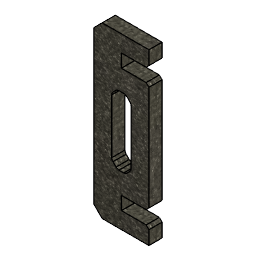
Ensamblaje Blimp CARTON PLUMA (Autodesk Fusion 360 archive; units mm, degrees)
design "SOPORTE INFERIOR"
Autodesk Fusion 360 part; units mm, degrees
(part 1 of 5)
sketch "Boceto1" plane through (0, 0, 0) normal (0, 1, 0) x (1, 0, 0)
  line L0 (3, 0) -> (20, 0)
  line L1 (20, 0) -> (20, -6)
  line L2 (20, -6) -> (10, -6)
  line L3 (10, -6) -> (10, -10.8)
  line L4 (10, -10.8) -> (20, -10.8)
  line L5 (20, -10.8) -> (20, -30.8)
  line L6 (20, -30.8) -> (0, -30.8)
  line L7 (0, -30.8) -> (0, -3)
  line L8 (3, 0) -> (0, -3)
  line L9 (6.5, -30.8) -> (6.5, -20.9213)
  line L10 (9.1213, -18.3) -> (10.8787, -18.3)
  line L11 (13.5, -20.9213) -> (13.5, -30.8)
  line L12 (6.9393, -19.8607) -> (8.0607, -18.7393)
  line L13 (11.9393, -18.7393) -> (13.0607, -19.8607)
  arc A0 (6.9393, -19.8607) -> (6.5, -20.9213) centre (8, -20.9213) ccw
  arc A1 (9.1213, -18.3) -> (8.0607, -18.7393) centre (9.1213, -19.8) ccw
  arc A2 (11.9393, -18.7393) -> (10.8787, -18.3) centre (10.8787, -19.8) ccw
  arc A3 (13.5, -20.9213) -> (13.0607, -19.8607) centre (12, -20.9213) ccw
  line L14 (13.5, -40.6787) -> (13.5, -30.8)
  arc A4 (13.0607, -41.7393) -> (13.5, -40.6787) centre (12, -40.6787) ccw
  line L15 (11.9393, -42.8607) -> (13.0607, -41.7393)
  arc A5 (10.8787, -43.3) -> (11.9393, -42.8607) centre (10.8787, -41.8) ccw
  line L16 (9.1213, -43.3) -> (10.8787, -43.3)
  arc A6 (8.0607, -42.8607) -> (9.1213, -43.3) centre (9.1213, -41.8) ccw
  line L17 (6.9393, -41.7393) -> (8.0607, -42.8607)
  arc A7 (6.5, -40.6787) -> (6.9393, -41.7393) centre (8, -40.6787) ccw
  line L18 (6.5, -30.8) -> (6.5, -40.6787)
  line L19 (20, -50.8) -> (20, -30.8)
  line L20 (0, -30.8) -> (0, -58.6)
  line L21 (10, -50.8) -> (20, -50.8)
  line L22 (20, -55.6) -> (10, -55.6)
  line L23 (10, -55.6) -> (10, -50.8)
  line L24 (20, -61.6) -> (20, -55.6)
  line L25 (3, -61.6) -> (20, -61.6)
  line L26 (3, -61.6) -> (0, -58.6)
  point P0 (6.5, -18.3)
  point P1 (13.5, -18.3)
  point P2 (6.5, -20.3)
  point P3 (8.5, -18.3)
  point P4 (11.5, -18.3)
  point P5 (13.5, -20.3)
  dimension "d1" = 4.8
  dimension "d2" = 40
  dimension "d3" = 6
  dimension "d4" = 20
  dimension "d5" = 10
  dimension "d6" = 3
  dimension "d7" = 3
  dimension "d8" = 7
  dimension "d10" = 7.5
  dimension "d11" = 6.5
  dimension "d12" = 2
  dimension "d13" = 2
  dimension "d14" = 2
  dimension "d15" = 2
  dimension "d16" = 1.5
  constraint horizontal L0
  constraint perpendicular L0 L1
  constraint perpendicular L1 L2
  constraint perpendicular L2 L3
  constraint perpendicular L1 L4
  constraint perpendicular L4 L5
  constraint perpendicular L1 L6
  constraint perpendicular L0 L7
  constraint coincident L1 L4.end
  constraint coincident origin L0
  constraint coincident origin L7
  constraint coincident L6 L9.start
  constraint perpendicular L6 L9
  constraint perpendicular L9 L10
  constraint coincident L6 L11.end
  constraint perpendicular L6 L11
  constraint coincident P0 L9
  constraint coincident P0 L10
  constraint coincident P1 L10
  constraint coincident P1 L11
  constraint coincident P2 L12
  constraint coincident L9 P2
  constraint tangent L12 A0
  constraint tangent L9 A0
  constraint coincident P3 L12
  constraint coincident L10 P3
  constraint tangent L12 A1
  constraint tangent L10 A1
  constraint equal A0 A1
  constraint coincident P4 L13
  constraint coincident L10 P4
  constraint tangent L13 A2
  constraint tangent L10 A2
  constraint equal A0 A2
  constraint coincident P5 L13
  constraint coincident L11 P5
  constraint tangent L13 A3
  constraint tangent L11 A3
  constraint equal A0 A3
  constraint symmetric L0.end L6 L24.start
  constraint symmetric L1.end L6 L22.start
  constraint symmetric L2.end L6 L22.end
  constraint symmetric L3.end L6 L21.start
  constraint symmetric L4.end L6 L19.start
  constraint symmetric L5.end L6 L19.end
  constraint symmetric L7.start L6 L20.start
  constraint symmetric L6 L0.start L25.start
  constraint symmetric L6 L7.end L20.end
  constraint symmetric L6 L9.start L18.start
  constraint symmetric L6 L11.end L14.end
  constraint symmetric L6 L12.start L17.start
  constraint symmetric L6 L9.end A7.start
  constraint symmetric L6 A0 A7
  constraint symmetric L6 L12.end A6.start
  constraint symmetric L6 L10.start L16.start
  constraint symmetric L6 A1 A6
  constraint symmetric L6 L13.start L15.start
  constraint symmetric L6 L10.end A5.start
  constraint symmetric L6 A2 A5
  constraint symmetric L6 L13.end A4.start
  constraint symmetric L6 L11.start L14.start
  constraint symmetric L6 A3 A4
  measures "d1" distance of L2.end L3.end
  measures "d3" distance of L0 L2
  measures "d4" distance of origin L0.end
  measures "d5" distance of L3 L7
  measures "d6" distance of origin L0.start
  measures "d7" distance of origin L7.end
  measures "d8" distance of P0 P1
  measures "d10" distance of L4 L10
  measures "d11" distance of L7 L9
  measures "d12" distance of P0 P2
  measures "d13" distance of P0 P3
  measures "d14" distance of P1 P4
  measures "d15" distance of P1 P5
  measures "d16" radius of A0
extrude "Extruir1" add sketch "Boceto1" along normal blind 4.8 contours L0 L1 L2 L3 L4 L5 L6 L7 L8 L9 L10 L11 L12 L13 A0 A1 A2 A3 | L6 L14 A4 L15 A5 L16 A6 L17 A7 L18 L19 L20 L21 L22 L23 L24 L25 L26
sketch "Boceto2" plane through (0, 0, 0) normal (0, -1, 0) x (1, 0, 0)
  arc A0 (6.5, 20.9213) -> (6.9393, 19.8607) centre (8, 20.9213) ccw
  line L0 (6.5, 20.9213) -> (6.5, 40.6787)
  arc A1 (6.9393, 41.7393) -> (6.5, 40.6787) centre (8, 40.6787) ccw
  line L1 (6.9393, 41.7393) -> (8.0607, 42.8607)
  arc A2 (9.1213, 43.3) -> (8.0607, 42.8607) centre (9.1213, 41.8) ccw
  line L2 (9.1213, 43.3) -> (10.8787, 43.3)
  arc A3 (11.9393, 42.8607) -> (10.8787, 43.3) centre (10.8787, 41.8) ccw
  line L3 (11.9393, 42.8607) -> (13.0607, 41.7393)
  arc A4 (13.5, 40.6787) -> (13.0607, 41.7393) centre (12, 40.6787) ccw
  line L4 (13.5, 40.6787) -> (13.5, 20.9213)
  arc A5 (13.0607, 19.8607) -> (13.5, 20.9213) centre (12, 20.9213) ccw
  line L5 (13.0607, 19.8607) -> (11.9393, 18.7393)
  arc A6 (10.8787, 18.3) -> (11.9393, 18.7393) centre (10.8787, 19.8) ccw
  line L6 (10.8787, 18.3) -> (9.1213, 18.3)
  arc A7 (8.0607, 18.7393) -> (9.1213, 18.3) centre (9.1213, 19.8) ccw
  line L7 (8.0607, 18.7393) -> (6.9393, 19.8607)
  line L8 (20, 55.6) -> (20, 61.6)
  line L9 (20, 61.6) -> (3, 61.6)
  line L10 (3, 61.6) -> (0, 58.6)
  line L11 (0, 58.6) -> (0, 3)
  line L12 (0, 3) -> (3, 0)
  line L13 (3, 0) -> (20, 0)
  line L14 (20, 0) -> (20, 6)
  line L15 (20, 6) -> (10, 6)
  line L16 (10, 6) -> (10, 10.8)
  line L17 (10, 10.8) -> (20, 10.8)
  line L18 (20, 10.8) -> (20, 50.8)
  line L19 (20, 50.8) -> (10, 50.8)
  line L20 (10, 50.8) -> (10, 55.6)
  line L21 (10, 55.6) -> (20, 55.6)
chamfer "Chaflán1" distance 1 angle 45 4 edges at (20, 2.4, 50.8) (20, 2.4, 55.6) (20, 2.4, 6) (20, 2.4, 10.8)
sketch "Boceto3" plane through (0, 0, 0) normal (0, -1, 0) x (1, 0, 0)
  arc A0 (6.5, 20.9213) -> (6.9393, 19.8607) centre (8, 20.9213) ccw
  line L0 (6.5, 20.9213) -> (6.5, 40.6787)
  arc A1 (6.9393, 41.7393) -> (6.5, 40.6787) centre (8, 40.6787) ccw
  line L1 (6.9393, 41.7393) -> (8.0607, 42.8607)
  arc A2 (9.1213, 43.3) -> (8.0607, 42.8607) centre (9.1213, 41.8) ccw
  line L2 (9.1213, 43.3) -> (10.8787, 43.3)
  arc A3 (11.9393, 42.8607) -> (10.8787, 43.3) centre (10.8787, 41.8) ccw
  line L3 (11.9393, 42.8607) -> (13.0607, 41.7393)
  arc A4 (13.5, 40.6787) -> (13.0607, 41.7393) centre (12, 40.6787) ccw
  line L4 (13.5, 40.6787) -> (13.5, 20.9213)
  arc A5 (13.0607, 19.8607) -> (13.5, 20.9213) centre (12, 20.9213) ccw
  line L5 (13.0607, 19.8607) -> (11.9393, 18.7393)
  arc A6 (10.8787, 18.3) -> (11.9393, 18.7393) centre (10.8787, 19.8) ccw
  line L6 (10.8787, 18.3) -> (9.1213, 18.3)
  arc A7 (8.0607, 18.7393) -> (9.1213, 18.3) centre (9.1213, 19.8) ccw
  line L7 (8.0607, 18.7393) -> (6.9393, 19.8607)
  line L8 (19, 10.8) -> (20, 11.8)
  line L9 (20, 11.8) -> (20, 49.8)
  line L10 (20, 49.8) -> (19, 50.8)
  line L11 (19, 50.8) -> (10, 50.8)
  line L12 (10, 50.8) -> (10, 55.6)
  line L13 (10, 55.6) -> (19, 55.6)
  line L14 (19, 55.6) -> (20, 56.6)
  line L15 (20, 56.6) -> (20, 61.6)
  line L16 (20, 61.6) -> (3, 61.6)
  line L17 (3, 61.6) -> (0, 58.6)
  line L18 (0, 58.6) -> (0, 3)
  line L19 (0, 3) -> (3, 0)
  line L20 (3, 0) -> (20, 0)
  line L21 (20, 0) -> (20, 5)
  line L22 (20, 5) -> (19, 6)
  line L23 (19, 6) -> (10, 6)
  line L24 (10, 6) -> (10, 10.8)
  line L25 (10, 10.8) -> (19, 10.8)
equation "d7 = d6"
equation "d13 = d12"
equation "d15 = d14"

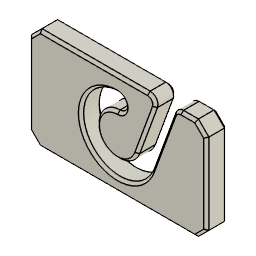
design "SOPORTE PEGADO"
Autodesk Fusion 360 part; units mm, degrees
sketch "Boceto1" plane through (0, 0, 0) normal (0, 1, 0) x (1, 0, 0)
  line L0 (-15, 9.5) -> (15, 9.5)
  line L1 (17, 7.5) -> (17, -8)
  line L2 (-17, -8) -> (-17, 7.5)
  arc A0 (0, -7) -> (0, -4) centre (0, -5.5) ccw
  line L3 (0, -1.75) -> (0, -22.5)
  line L4 (3.7588, 1.3681) -> (7.1637, -7.987)
  line L5 (6.5778, 2.3941) -> (10.7297, -9.013)
  arc A1 (6.5778, 2.3941) -> (0, -7) centre (0, 0) ccw
  arc A2 (3.7588, 1.3681) -> (0, -4) centre (0, 0) ccw
  line L6 (15, -10) -> (12.1393, -10)
  line L7 (5.7542, -10) -> (-15, -10)
  line L8 (-17, -8) -> (-15, -10)
  line L9 (-15, 9.5) -> (-17, 7.5)
  line L10 (15, 9.5) -> (17, 7.5)
  line L11 (17, -8) -> (15, -10)
  arc A3 (5.7542, -10) -> (7.1637, -7.987) centre (5.7542, -8.5) ccw
  arc A4 (10.7297, -9.013) -> (12.1393, -10) centre (12.1393, -8.5) ccw
  point P0 (-17, 9.5)
  point P1 (17, 9.5)
  point P2 (17, -10)
  point P3 (-17, -10)
  dimension "d1" = 8
  dimension "d2" = 14
  dimension "d4" = 10
  dimension "d5" = 9.5
  dimension "d7" = 1.5
  dimension "d8" = 20
  dimension "d9" = 34
  dimension "d10" = 17
  dimension "d11" = 2
  dimension "d12" = 2
  dimension "d13" = 2
  dimension "d14" = 2
  dimension "d15" = 2
  dimension "d16" = 2
  dimension "d17" = 2
  dimension "d18" = 2
  dimension "d19" = 1.5
  constraint coincident A1.centre A2.centre
  constraint concentric A1 A2
  constraint horizontal L0
  constraint vertical L1
  constraint horizontal L6
  constraint vertical L2
  constraint coincident A0.start L3
  constraint coincident A0.end L3
  constraint tangent L4 A2
  constraint parallel L4 L5
  constraint tangent L5 A1
  constraint collinear L6 L7
  constraint coincident P3 L2
  constraint coincident P3 L7
  constraint coincident P0 L0
  constraint coincident P0 L2
  constraint coincident P1 L0
  constraint coincident P1 L1
  constraint coincident P2 L1
  constraint coincident P2 L6
  constraint tangent L4 A3
  constraint tangent L7 A3
  constraint tangent L5 A4
  constraint tangent L6 A4
  constraint equal A3 A4
  measures "d1" diameter of A2
  measures "d2" diameter of A1
  measures "d4" distance of A1.centre L7
  measures "d5" distance of A1.centre L0
  measures "d7" radius of A0
  measures "d8" angle of L3 L4
  measures "d9" distance of L1 L2
  measures "d10" distance of A1.centre L2
  measures "d11" distance of P3 L2.start
  measures "d12" distance of P3 L7.end
  measures "d13" distance of P0 L0.start
  measures "d14" distance of P0 L2.end
  measures "d15" distance of P1 L0.end
  measures "d16" distance of P1 L1.start
  measures "d17" distance of P2 L1.end
  measures "d18" distance of P2 L6.start
  measures "d19" radius of A3
extrude "Extruir1" add sketch "Boceto1" along normal blind 4 contours L0 L1 L2 L3 L5 A1 L6 L7 L8 L9 L10 L11 A4 | A0 L3 L4 A2 L7 A3
chamfer "Chaflán1" distance 0.5 angle 45 2 faces at (13.5259, 0, -0.6314) (13.5259, 4, -0.6314)
equation "d10 = d9 / 2"
equation "d12 = d11"
equation "d14 = d13"
equation "d16 = d15"
equation "d18 = d17"

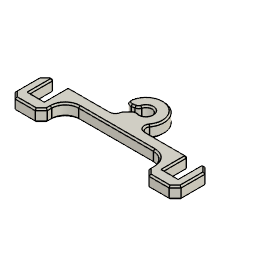
design "SOPORTE IMPRESO GLOBO"
Autodesk Fusion 360 part; units mm, degrees
sketch "Boceto1" plane through (0, 0, 0) normal (0, 0, 1) x (1, 0, 0)
  circle A0 centre (0, 0) radius 2
  circle A1 centre (0, 0) radius 6
  line L0 (-20, -6) -> (-20, -14)
  line L1 (-20, -14) -> (-24.75, -14)
  line L2 (-24.75, -14) -> (-24.75, -6)
  line L3 (-24.75, -6) -> (-27.75, -6)
  line L4 (-27.75, -6) -> (-27.75, -18)
  line L5 (-27.75, -18) -> (-17, -18)
  line L6 (0, -18) -> (0, -6)
  line L7 (-17, -6) -> (-17, -10)
  line L8 (-20, -6) -> (-17, -6)
  line L9 (-4.2426, -4.2426) -> (-4.2426, -6)
  line L10 (-5.9088, -1.0419) -> (-1.9696, -0.3473)
  line L11 (-4.2426, -4.2426) -> (-1.4142, -1.4142)
  line L12 (-24.75, -14) -> (-24.75, 6) construction
  line L13 (0, 6) -> (-24.75, 6) construction
  line L14 (-17, -6) -> (-4.2426, -6)
  line L15 (-17, -10) -> (0, -10)
  line L16 (-17, -10) -> (-17, -18)
  line L17 (24.75, -14) -> (24.75, -6)
  line L18 (24.75, -6) -> (27.75, -6)
  line L19 (27.75, -6) -> (27.75, -18)
  line L20 (27.75, -18) -> (17, -18)
  line L21 (20, -14) -> (24.75, -14)
  line L22 (20, -6) -> (20, -14)
  line L23 (20, -6) -> (17, -6)
  line L24 (17, -6) -> (4.2426, -6)
  line L25 (17, -10) -> (0, -10)
  line L26 (17, -10) -> (17, -18)
  line L27 (4.2426, -4.2426) -> (4.2426, -6)
  dimension "d1" = 4
  dimension "d2" = 4
  dimension "d3" = 4.75
  dimension "d4" = 3
  dimension "d5" = 4
  dimension "d6" = 8
  dimension "d7" = 45
  dimension "d8" = 35
  dimension "d9" = 20
  dimension "d11" = 3
  dimension "d12" = 4
  dimension "d22" = 40
  constraint coincident A0.centre A1.centre
  constraint perpendicular L0 L1
  constraint perpendicular L1 L2
  constraint perpendicular L2 L3
  constraint perpendicular L3 L4
  constraint perpendicular L2 L5
  constraint coincident A1 L6.end
  constraint perpendicular L5 L6
  constraint coincident A0.centre L6
  constraint perpendicular L7 L8
  constraint coincident L2.end L8
  constraint horizontal L8
  constraint horizontal L5
  constraint coincident A1 L9.start
  constraint perpendicular L8 L9
  constraint coincident A1 L10.start
  constraint coincident A0 L10.end
  constraint coincident A0.centre L10
  constraint coincident A0 L11.end
  constraint coincident A0.centre L11
  constraint coincident A1 L13.start
  constraint perpendicular L12 L13
  constraint tangent A1 L13
  constraint coincident L12.end L13.end
  constraint coincident L1 L2.start
  constraint vertical L12
  constraint coincident L1.end L2.start
  constraint perpendicular L9 L14
  constraint perpendicular L9 L15
  constraint perpendicular L5 L16
  constraint coincident L6 L15.end
  constraint symmetric L0.start L6 L22.start
  constraint symmetric L0.end L6 L21.start
  constraint symmetric L1.end L6 L17.start
  constraint symmetric L2.end L6 L17.end
  constraint symmetric L3.end L6 L18.end
  constraint symmetric L4.end L6 L19.end
  constraint symmetric L6 L7.start L23.end
  constraint symmetric L6 L9.start L27.start
  constraint symmetric L6 L9.end L24.end
  constraint symmetric L6 L7.end L25.start
  constraint symmetric L6 L15.end L25.end
  constraint symmetric L6 L5.end L20.end
  measures "d1" diameter of A0
  measures "d2" distance of A0
  measures "d3" distance of L0.end L1.end
  measures "d4" distance of L2.end L3.end
  measures "d5" distance of L1 L5
  measures "d6" distance of L1.end L2.end
  measures "d7" angle of L6 L11
  measures "d8" angle of L10 L11
  measures "d9" distance of L1.end L12.end
  measures "d11" distance of L0.start L7.start
  measures "d12" distance of L14 L15
extrude "Extruir1" add sketch "Boceto1" along normal blind 4 contours A0 A1 L10 L11 | A1 L6 L7 L9 L14 L15 | A1 L6 L17 L18 L19 L20 L21 L22 L23 L24 L25 L26 L27 | L0 L1 L2 L3 L4 L5 L7 L8 L16 picked at (-4.6252, -0.5238)
fillet "Empalme1" radius 4.5 2 edges at (-17, -10, 2) (17, -10, 2)
fillet "Empalme2" radius 1.5 7 edges at (-1.4142, -1.4142, 2) (-1.9696, -0.3473, 2) (-5.9088, -1.0419, 2) (-4.2426, -4.2426, 2) (-4.2426, -6, 2) (4.2426, -6, 2) (4.2426, -4.2426, 2)
chamfer "Chaflán1" distance 0.5 angle 45 4 edges at (-20, -6, 2) (-24.75, -6, 2) (20, -6, 2) (24.75, -6, 2)
chamfer "Chaflán2" distance 2 angle 45 6 edges at (27.75, -6, 2) (27.75, -18, 2) (17, -18, 2) (-17, -18, 2) (-27.75, -18, 2) (-27.75, -6, 2)
chamfer "Chaflán3" distance 0.5 angle 45 2 faces at (-12.5735, -7.3333, 4) (-12.5735, -7.3333, 0)
equation "d11 = d4"

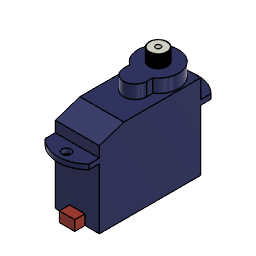
design "MINI SERVO"
Autodesk Fusion 360 part; units mm, degrees
sketch "Boceto1" plane through (0, 0, 0) normal (0, 0, 1) x (1, 0, 0)
  line L0 (0, 0) -> (8.6, 0)
  line L1 (8.6, 0) -> (8.6, 19.8)
  line L2 (8.6, 19.8) -> (0, 19.8)
  line L3 (0, 19.8) -> (0, 0)
  dimension "d1" = 8.6
  dimension "d2" = 19.8
  constraint horizontal L0
  constraint vertical L1
  constraint horizontal L2
  constraint vertical L3
  constraint coincident L0.start L3.end
  measures "d1" distance of L0.start L0.end
  measures "d2" distance of L0.start L2.end
extrude "Extruir1" add sketch "Boceto1" along normal blind 11.85 makes body 1
sketch "Boceto2" plane through (0, 0, 0) normal (0, -1, 0) x (1, 0, 0)
  line L0 (0, 0) -> (8.6, 0)
  line L1 (8.6, 0) -> (8.6, 11.85)
  line L2 (8.6, 11.85) -> (0, 11.85)
  line L3 (0, 11.85) -> (0, 0)
  line L4 (2.8, 0) -> (5.8, 0)
  line L5 (5.8, 0) -> (5.8, 2)
  line L6 (5.8, 2) -> (2.8, 2)
  line L7 (2.8, 2) -> (2.8, 0)
  dimension "d5" = 3
  dimension "d6" = 2
  dimension "d7" = 2.8
  dimension "d8" = 8.6
  constraint horizontal L4
  constraint vertical L5
  constraint horizontal L6
  constraint vertical L7
  constraint coincident L0 L4.start
  measures "d5" distance of L4.start L4.end
  measures "d6" distance of L4.start L6.end
  measures "d7" distance of L0.start L4.start
  measures "d8" distance of L1.end L2.end
extrude "Extruir2" add sketch "Boceto2" along normal blind 2 separate body contours L0 L4 L5 L6 L7 makes body 2
sketch "Boceto3" plane through (0, 0, 11.85) normal (0, 0, 1) x (-1, 0, 0)
  line L0 (0, -19.8) -> (0, 0)
  line L1 (0, 0) -> (-8.6, 0)
  line L2 (-8.6, 0) -> (-8.6, -19.8)
  line L3 (-8.6, -19.8) -> (0, -19.8)
  line L4 (0, -23.6) -> (-8.6, -23.6)
  line L5 (-8.6, -23.6) -> (-8.6, 3.8)
  line L6 (-8.6, 3.8) -> (0, 3.8)
  line L7 (0, 3.8) -> (0, -23.6)
  circle A0 centre (-4.3, -21.9) radius 0.875
  line L8 (-8.6, -9.9) -> (0, -9.9)
  line L9 (-4.3, -19.8) -> (-4.3, -23.6) construction
  arc A1 (-4.3, -23.6) -> (0, -21.8) centre (-4.3, -17.5639) ccw
  arc A2 (-8.6, -21.8) -> (-4.3, -23.6) centre (-4.3, -17.5639) ccw
  arc A3 (0, 2) -> (-4.3, 3.8) centre (-4.3, -2.2361) ccw
  arc A4 (-4.3, 3.8) -> (-8.6, 2) centre (-4.3, -2.2361) ccw
  circle A5 centre (-4.3, 2.1) radius 0.875
  dimension "d11" = 27.4
  dimension "d12" = 3.8
  dimension "d13" = 1.75
  dimension "d14" = 2.1
  dimension "d15" = 2
  constraint horizontal L4
  constraint vertical L5
  constraint horizontal L6
  constraint vertical L7
  constraint midpoint L5 L8.start
  constraint midpoint L7 L8.end
  constraint coincident L0.start L7
  constraint coincident L2.end L5
  constraint midpoint L3 L9.start
  constraint midpoint L4 L9.end
  constraint coincident A0.centre L9
  constraint tangent L4 A1
  constraint coincident L7 A1.end
  constraint symmetric A1.start L9 A2.end
  constraint symmetric L9 A1.end A2.start
  constraint symmetric L9 A1 A2
  constraint symmetric A0 L8 A5
  constraint symmetric L8 L9.end A3.end
  constraint symmetric L8 A1.end A3.start
  constraint symmetric L8 A1 A3
  constraint symmetric L8 A2.start A4.end
  constraint symmetric L8 A2 A4
  measures "d11" distance of L4.end L5.end
  measures "d12" distance of L3 L4
  measures "d13" diameter of A0
  measures "d14" distance of L3 A0.centre
  measures "d15" distance of L0.start A1.end
extrude "Extruir3" add sketch "Boceto3" along normal blind 0.95 contours L0 L2 L3 L5 L7 L8 | L3 L5 L7 A1 A2 | L0 L1 L2 L5 L7 L8 | L1 L5 L7 A3 A4 bodies 1
sketch "Boceto4" plane through (0, 0, 12.8) normal (0, 0, 1) x (-1, 0, 0)
  circle A0 centre (-4.3, 2.1) radius 0.875
  circle A1 centre (-4.3, -21.9) radius 0.875
  arc A2 (0, 2) -> (-8.6, 2) centre (-4.3, -2.2361) ccw
  line L0 (-8.6, 2) -> (-8.6, -21.8)
  arc A3 (-8.6, -21.8) -> (0, -21.8) centre (-4.3, -17.5639) ccw
  line L1 (0, -21.8) -> (0, 2)
  line L2 (0, 0) -> (-8.6, 0)
  line L3 (-8.6, 0) -> (-8.6, -19.8)
  line L4 (-8.6, -19.8) -> (0, -19.8)
  line L5 (0, -19.8) -> (0, 0)
  dimension "d18" = 19.8
  constraint horizontal L2
  constraint vertical L3
  constraint horizontal L4
  constraint vertical L5
  constraint coincident L0 L3.end
  constraint coincident L2.start L5.end
  measures "d18" distance of L2.end L3.end
extrude "Extruir4" add sketch "Boceto4" along normal blind 3.7 contours L0 L1 L2 L3 L4 L5 bodies 1
sketch "Boceto5" plane through (0, 0, 16.5) normal (0, 0, 1) x (-1, 0, 0)
  line L0 (0, -19.8) -> (0, 0)
  line L1 (0, 0) -> (-8.6, 0)
  line L2 (-8.6, 0) -> (-8.6, -19.8)
  line L3 (-8.6, -19.8) -> (0, -19.8)
  circle A0 centre (-4.3, -15.8) radius 4
  line L4 (-4.3, -19.8) -> (-4.3, 0)
  line L5 (-2.05, -11.3) -> (-2.05, -12.4928)
  line L6 (-6.55, -11.3) -> (-6.55, -12.4928)
  arc A1 (-2.05, -11.3) -> (-6.55, -11.3) centre (-4.3, -11.3) ccw
  dimension "d21" = 8
  dimension "d22" = 4.5
  dimension "d23" = 4.5
  constraint tangent L3 A0
  constraint midpoint L3 L4.start
  constraint midpoint L1 L4.end
  constraint coincident A0.centre L4
  constraint coincident A0 L5.end
  constraint tangent L5 A1
  constraint parallel L4 L5
  constraint coincident A0 L6.end
  constraint tangent L6 A1
  constraint parallel L4 L6
  constraint coincident L4 A1.centre
  measures "d21" diameter of A0
  measures "d22" diameter of A1
  measures "d23" distance of A0.centre A1.centre
extrude "Extruir5" add sketch "Boceto5" along normal blind 2.6 contours A0 L4 | A0 L4 | A0 L4 L6 A1 | A0 L4 L5 A1 bodies 1
chamfer "Chaflán1" distance 4.8 distance2 1.6 1 edges at (4.3, 0, 16.5) measured on face at (4.356, 3.0188, 16.5) on bodies 1
sketch "Boceto6" plane through (0, 0, 19.1) normal (0, 0, 1) x (-1, 0, 0)
  arc A0 (-2.05, -11.3) -> (-6.55, -11.3) centre (-4.3, -11.3) ccw
  line L0 (-6.55, -11.3) -> (-6.55, -12.4928)
  arc A1 (-6.55, -12.4928) -> (-2.05, -12.4928) centre (-4.3, -15.8) ccw
  line L1 (-2.05, -12.4928) -> (-2.05, -11.3)
  circle A2 centre (-4.3, -15.8) radius 1.75
  circle A3 centre (-4.3, -15.8) radius 0.5
  line L2 (-4.2713, -17.5498) -> (-4.28, -17.5005)
  line L3 (-4.28, -17.5005) -> (-4.32, -17.5005)
  line L4 (-4.32, -17.5005) -> (-4.3287, -17.5498)
  line L5 (-4.3, -17.5005) -> (-4.3, -15.8) construction
  line L6 (-4.2132, -17.4984) -> (-4.2188, -17.5481)
  line L7 (-4.1733, -17.4959) -> (-4.2132, -17.4984)
  line L8 (-4.1615, -17.5445) -> (-4.1733, -17.4959)
  line L9 (-4.1067, -17.4896) -> (-4.1092, -17.5396)
  line L10 (-4.067, -17.4846) -> (-4.1067, -17.4896)
  line L11 (-4.0522, -17.5324) -> (-4.067, -17.4846)
  line L12 (-4.001, -17.4742) -> (-4.0003, -17.5241)
  line L13 (-3.9617, -17.4667) -> (-4.001, -17.4742)
  line L14 (-3.944, -17.5134) -> (-3.9617, -17.4667)
  line L15 (-3.8965, -17.4521) -> (-3.8926, -17.5019)
  line L16 (-3.8577, -17.4421) -> (-3.8965, -17.4521)
  line L17 (-3.8371, -17.4877) -> (-3.8577, -17.4421)
  line L18 (-3.7935, -17.4235) -> (-3.7866, -17.473)
  line L19 (-3.7555, -17.4111) -> (-3.7935, -17.4235)
  line L20 (-3.732, -17.4553) -> (-3.7555, -17.4111)
  line L21 (-3.6926, -17.3885) -> (-3.6825, -17.4374)
  line L22 (-3.6554, -17.3737) -> (-3.6926, -17.3885)
  line L23 (-3.6292, -17.4163) -> (-3.6554, -17.3737)
  line L24 (-3.594, -17.3472) -> (-3.5809, -17.3954)
  line L25 (-3.5579, -17.3302) -> (-3.594, -17.3472)
  line L26 (-3.529, -17.371) -> (-3.5579, -17.3302)
  line L27 (-3.4983, -17.2998) -> (-3.4822, -17.3471)
  line L28 (-3.4632, -17.2805) -> (-3.4983, -17.2998)
  line L29 (-3.4319, -17.3195) -> (-3.4632, -17.2805)
  line L30 (-3.4057, -17.2465) -> (-3.3866, -17.2927)
  line L31 (-3.3719, -17.2251) -> (-3.4057, -17.2465)
  line L32 (-3.3382, -17.262) -> (-3.3719, -17.2251)
  line L33 (-3.3166, -17.1875) -> (-3.2947, -17.2324)
  line L34 (-3.2843, -17.164) -> (-3.3166, -17.1875)
  line L35 (-3.2483, -17.1987) -> (-3.2843, -17.164)
  line L36 (-3.2315, -17.123) -> (-3.2068, -17.1665)
  line L37 (-3.2006, -17.0975) -> (-3.2315, -17.123)
  line L38 (-3.1626, -17.1299) -> (-3.2006, -17.0975)
  line L39 (-3.1505, -17.0533) -> (-3.1231, -17.0952)
  line L40 (-3.1213, -17.0259) -> (-3.1505, -17.0533)
  line L41 (-3.0813, -17.0559) -> (-3.1213, -17.0259)
  line L42 (-3.0741, -16.9787) -> (-3.0441, -17.0187)
  line L43 (-3.0467, -16.9495) -> (-3.0741, -16.9787)
  line L44 (-3.0048, -16.9769) -> (-3.0467, -16.9495)
  line L45 (-3.0025, -16.8994) -> (-2.9701, -16.9374)
  line L46 (-2.977, -16.8685) -> (-3.0025, -16.8994)
  line L47 (-2.9335, -16.8932) -> (-2.977, -16.8685)
  line L48 (-2.936, -16.8157) -> (-2.9013, -16.8517)
  line L49 (-2.9125, -16.7834) -> (-2.936, -16.8157)
  line L50 (-2.8676, -16.8053) -> (-2.9125, -16.7834)
  line L51 (-2.8749, -16.7281) -> (-2.838, -16.7618)
  line L52 (-2.8535, -16.6943) -> (-2.8749, -16.7281)
  line L53 (-2.8073, -16.7134) -> (-2.8535, -16.6943)
  line L54 (-2.8195, -16.6368) -> (-2.7805, -16.6681)
  line L55 (-2.8002, -16.6017) -> (-2.8195, -16.6368)
  line L56 (-2.7529, -16.6178) -> (-2.8002, -16.6017)
  line L57 (-2.7698, -16.5421) -> (-2.729, -16.571)
  line L58 (-2.7528, -16.506) -> (-2.7698, -16.5421)
  line L59 (-2.7046, -16.5191) -> (-2.7528, -16.506)
  line L60 (-2.7263, -16.4446) -> (-2.6837, -16.4708)
  line L61 (-2.7115, -16.4074) -> (-2.7263, -16.4446)
  line L62 (-2.6626, -16.4175) -> (-2.7115, -16.4074)
  line L63 (-2.6889, -16.3445) -> (-2.6447, -16.368)
  line L64 (-2.6765, -16.3065) -> (-2.6889, -16.3445)
  line L65 (-2.627, -16.3134) -> (-2.6765, -16.3065)
  line L66 (-2.6579, -16.2423) -> (-2.6123, -16.2629)
  line L67 (-2.6479, -16.2035) -> (-2.6579, -16.2423)
  line L68 (-2.5981, -16.2074) -> (-2.6479, -16.2035)
  line L69 (-2.6333, -16.1383) -> (-2.5866, -16.156)
  line L70 (-2.6258, -16.099) -> (-2.6333, -16.1383)
  line L71 (-2.5759, -16.0997) -> (-2.6258, -16.099)
  line L72 (-2.6154, -16.033) -> (-2.5676, -16.0478)
  line L73 (-2.6104, -15.9933) -> (-2.6154, -16.033)
  line L74 (-2.5604, -15.9908) -> (-2.6104, -15.9933)
  line L75 (-2.6041, -15.9267) -> (-2.5555, -15.9385)
  line L76 (-2.6016, -15.8868) -> (-2.6041, -15.9267)
  line L77 (-2.5519, -15.8812) -> (-2.6016, -15.8868)
  line L78 (-2.5995, -15.82) -> (-2.5502, -15.8287)
  line L79 (-2.5995, -15.78) -> (-2.5995, -15.82)
  line L80 (-2.5502, -15.7713) -> (-2.5995, -15.78)
  line L81 (-2.6016, -15.7132) -> (-2.5519, -15.7188)
  line L82 (-2.6041, -15.6733) -> (-2.6016, -15.7132)
  line L83 (-2.5555, -15.6615) -> (-2.6041, -15.6733)
  line L84 (-2.6104, -15.6067) -> (-2.5604, -15.6092)
  line L85 (-2.6154, -15.567) -> (-2.6104, -15.6067)
  line L86 (-2.5676, -15.5522) -> (-2.6154, -15.567)
  line L87 (-2.6258, -15.501) -> (-2.5759, -15.5003)
  line L88 (-2.6333, -15.4617) -> (-2.6258, -15.501)
  line L89 (-2.5866, -15.444) -> (-2.6333, -15.4617)
  line L90 (-2.6479, -15.3965) -> (-2.5981, -15.3926)
  line L91 (-2.6579, -15.3577) -> (-2.6479, -15.3965)
  line L92 (-2.6123, -15.3371) -> (-2.6579, -15.3577)
  line L93 (-2.6765, -15.2935) -> (-2.627, -15.2866)
  line L94 (-2.6889, -15.2555) -> (-2.6765, -15.2935)
  line L95 (-2.6447, -15.232) -> (-2.6889, -15.2555)
  line L96 (-2.7115, -15.1926) -> (-2.6626, -15.1825)
  line L97 (-2.7263, -15.1554) -> (-2.7115, -15.1926)
  line L98 (-2.6837, -15.1292) -> (-2.7263, -15.1554)
  line L99 (-2.7528, -15.094) -> (-2.7046, -15.0809)
  line L100 (-2.7698, -15.0579) -> (-2.7528, -15.094)
  line L101 (-2.729, -15.029) -> (-2.7698, -15.0579)
  line L102 (-2.8002, -14.9983) -> (-2.7529, -14.9822)
  line L103 (-2.8195, -14.9632) -> (-2.8002, -14.9983)
  line L104 (-2.7805, -14.9319) -> (-2.8195, -14.9632)
  line L105 (-2.8535, -14.9057) -> (-2.8073, -14.8866)
  line L106 (-2.8749, -14.8719) -> (-2.8535, -14.9057)
  line L107 (-2.838, -14.8382) -> (-2.8749, -14.8719)
  line L108 (-2.9125, -14.8166) -> (-2.8676, -14.7947)
  line L109 (-2.936, -14.7843) -> (-2.9125, -14.8166)
  line L110 (-2.9013, -14.7483) -> (-2.936, -14.7843)
  line L111 (-2.977, -14.7315) -> (-2.9335, -14.7068)
  line L112 (-3.0025, -14.7006) -> (-2.977, -14.7315)
  line L113 (-2.9701, -14.6626) -> (-3.0025, -14.7006)
  line L114 (-3.0467, -14.6505) -> (-3.0048, -14.6231)
  line L115 (-3.0741, -14.6213) -> (-3.0467, -14.6505)
  line L116 (-3.0441, -14.5813) -> (-3.0741, -14.6213)
  line L117 (-3.1213, -14.5741) -> (-3.0813, -14.5441)
  line L118 (-3.1505, -14.5467) -> (-3.1213, -14.5741)
  line L119 (-3.1231, -14.5048) -> (-3.1505, -14.5467)
  line L120 (-3.2006, -14.5025) -> (-3.1626, -14.4701)
  line L121 (-3.2315, -14.477) -> (-3.2006, -14.5025)
  line L122 (-3.2068, -14.4335) -> (-3.2315, -14.477)
  line L123 (-3.2843, -14.436) -> (-3.2483, -14.4013)
  line L124 (-3.3166, -14.4125) -> (-3.2843, -14.436)
  line L125 (-3.2947, -14.3676) -> (-3.3166, -14.4125)
  line L126 (-3.3719, -14.3749) -> (-3.3382, -14.338)
  line L127 (-3.4057, -14.3535) -> (-3.3719, -14.3749)
  line L128 (-3.3866, -14.3073) -> (-3.4057, -14.3535)
  line L129 (-3.4632, -14.3195) -> (-3.4319, -14.2805)
  line L130 (-3.4983, -14.3002) -> (-3.4632, -14.3195)
  line L131 (-3.4822, -14.2529) -> (-3.4983, -14.3002)
  line L132 (-3.5579, -14.2698) -> (-3.529, -14.229)
  line L133 (-3.594, -14.2528) -> (-3.5579, -14.2698)
  line L134 (-3.5809, -14.2046) -> (-3.594, -14.2528)
  line L135 (-3.6554, -14.2263) -> (-3.6292, -14.1837)
  line L136 (-3.6926, -14.2115) -> (-3.6554, -14.2263)
  line L137 (-3.6825, -14.1626) -> (-3.6926, -14.2115)
  line L138 (-3.7555, -14.1889) -> (-3.732, -14.1447)
  line L139 (-3.7935, -14.1765) -> (-3.7555, -14.1889)
  line L140 (-3.7866, -14.127) -> (-3.7935, -14.1765)
  line L141 (-3.8577, -14.1579) -> (-3.8371, -14.1123)
  line L142 (-3.8965, -14.1479) -> (-3.8577, -14.1579)
  line L143 (-3.8926, -14.0981) -> (-3.8965, -14.1479)
  line L144 (-3.9617, -14.1333) -> (-3.944, -14.0866)
  line L145 (-4.001, -14.1258) -> (-3.9617, -14.1333)
  line L146 (-4.0003, -14.0759) -> (-4.001, -14.1258)
  line L147 (-4.067, -14.1154) -> (-4.0522, -14.0676)
  line L148 (-4.1067, -14.1104) -> (-4.067, -14.1154)
  line L149 (-4.1092, -14.0604) -> (-4.1067, -14.1104)
  line L150 (-4.1733, -14.1041) -> (-4.1615, -14.0555)
  line L151 (-4.2132, -14.1016) -> (-4.1733, -14.1041)
  line L152 (-4.2188, -14.0519) -> (-4.2132, -14.1016)
  line L153 (-4.28, -14.0995) -> (-4.2713, -14.0502)
  line L154 (-4.32, -14.0995) -> (-4.28, -14.0995)
  line L155 (-4.3287, -14.0502) -> (-4.32, -14.0995)
  line L156 (-4.3868, -14.1016) -> (-4.3812, -14.0519)
  line L157 (-4.4267, -14.1041) -> (-4.3868, -14.1016)
  line L158 (-4.4385, -14.0555) -> (-4.4267, -14.1041)
  line L159 (-4.4933, -14.1104) -> (-4.4908, -14.0604)
  line L160 (-4.533, -14.1154) -> (-4.4933, -14.1104)
  line L161 (-4.5478, -14.0676) -> (-4.533, -14.1154)
  line L162 (-4.599, -14.1258) -> (-4.5997, -14.0759)
  line L163 (-4.6383, -14.1333) -> (-4.599, -14.1258)
  line L164 (-4.656, -14.0866) -> (-4.6383, -14.1333)
  line L165 (-4.7035, -14.1479) -> (-4.7074, -14.0981)
  line L166 (-4.7423, -14.1579) -> (-4.7035, -14.1479)
  line L167 (-4.7629, -14.1123) -> (-4.7423, -14.1579)
  line L168 (-4.8065, -14.1765) -> (-4.8134, -14.127)
  line L169 (-4.8445, -14.1889) -> (-4.8065, -14.1765)
  line L170 (-4.868, -14.1447) -> (-4.8445, -14.1889)
  line L171 (-4.9074, -14.2115) -> (-4.9175, -14.1626)
  line L172 (-4.9446, -14.2263) -> (-4.9074, -14.2115)
  line L173 (-4.9708, -14.1837) -> (-4.9446, -14.2263)
  line L174 (-5.006, -14.2528) -> (-5.0191, -14.2046)
  line L175 (-5.0421, -14.2698) -> (-5.006, -14.2528)
  line L176 (-5.071, -14.229) -> (-5.0421, -14.2698)
  line L177 (-5.1017, -14.3002) -> (-5.1178, -14.2529)
  line L178 (-5.1368, -14.3195) -> (-5.1017, -14.3002)
  line L179 (-5.1681, -14.2805) -> (-5.1368, -14.3195)
  line L180 (-5.1943, -14.3535) -> (-5.2134, -14.3073)
  line L181 (-5.2281, -14.3749) -> (-5.1943, -14.3535)
  line L182 (-5.2618, -14.338) -> (-5.2281, -14.3749)
  line L183 (-5.2834, -14.4125) -> (-5.3053, -14.3676)
  line L184 (-5.3157, -14.436) -> (-5.2834, -14.4125)
  line L185 (-5.3517, -14.4013) -> (-5.3157, -14.436)
  line L186 (-5.3685, -14.477) -> (-5.3932, -14.4335)
  line L187 (-5.3994, -14.5025) -> (-5.3685, -14.477)
  line L188 (-5.4374, -14.4701) -> (-5.3994, -14.5025)
  line L189 (-5.4495, -14.5467) -> (-5.4769, -14.5048)
  line L190 (-5.4787, -14.5741) -> (-5.4495, -14.5467)
  line L191 (-5.5187, -14.5441) -> (-5.4787, -14.5741)
  line L192 (-5.5259, -14.6213) -> (-5.5559, -14.5813)
  line L193 (-5.5533, -14.6505) -> (-5.5259, -14.6213)
  line L194 (-5.5952, -14.6231) -> (-5.5533, -14.6505)
  line L195 (-5.5975, -14.7006) -> (-5.6299, -14.6626)
  line L196 (-5.623, -14.7315) -> (-5.5975, -14.7006)
  line L197 (-5.6665, -14.7068) -> (-5.623, -14.7315)
  line L198 (-5.664, -14.7843) -> (-5.6987, -14.7483)
  line L199 (-5.6875, -14.8166) -> (-5.664, -14.7843)
  line L200 (-5.7324, -14.7947) -> (-5.6875, -14.8166)
  line L201 (-5.7251, -14.8719) -> (-5.762, -14.8382)
  line L202 (-5.7465, -14.9057) -> (-5.7251, -14.8719)
  line L203 (-5.7927, -14.8866) -> (-5.7465, -14.9057)
  line L204 (-5.7805, -14.9632) -> (-5.8195, -14.9319)
  line L205 (-5.7998, -14.9983) -> (-5.7805, -14.9632)
  line L206 (-5.8471, -14.9822) -> (-5.7998, -14.9983)
  line L207 (-5.8302, -15.0579) -> (-5.871, -15.029)
  line L208 (-5.8472, -15.094) -> (-5.8302, -15.0579)
  line L209 (-5.8954, -15.0809) -> (-5.8472, -15.094)
  line L210 (-5.8737, -15.1554) -> (-5.9163, -15.1292)
  line L211 (-5.8885, -15.1926) -> (-5.8737, -15.1554)
  line L212 (-5.9374, -15.1825) -> (-5.8885, -15.1926)
  line L213 (-5.9111, -15.2555) -> (-5.9553, -15.232)
  line L214 (-5.9235, -15.2935) -> (-5.9111, -15.2555)
  line L215 (-5.973, -15.2866) -> (-5.9235, -15.2935)
  line L216 (-5.9421, -15.3577) -> (-5.9877, -15.3371)
  line L217 (-5.9521, -15.3965) -> (-5.9421, -15.3577)
  line L218 (-6.0019, -15.3926) -> (-5.9521, -15.3965)
  line L219 (-5.9667, -15.4617) -> (-6.0134, -15.444)
  line L220 (-5.9742, -15.501) -> (-5.9667, -15.4617)
  line L221 (-6.0241, -15.5003) -> (-5.9742, -15.501)
  line L222 (-5.9846, -15.567) -> (-6.0324, -15.5522)
  line L223 (-5.9896, -15.6067) -> (-5.9846, -15.567)
  line L224 (-6.0396, -15.6092) -> (-5.9896, -15.6067)
  line L225 (-5.9959, -15.6733) -> (-6.0445, -15.6615)
  line L226 (-5.9984, -15.7132) -> (-5.9959, -15.6733)
  line L227 (-6.0481, -15.7188) -> (-5.9984, -15.7132)
  line L228 (-6.0005, -15.78) -> (-6.0498, -15.7713)
  line L229 (-6.0005, -15.82) -> (-6.0005, -15.78)
  line L230 (-6.0498, -15.8287) -> (-6.0005, -15.82)
  line L231 (-5.9984, -15.8868) -> (-6.0481, -15.8812)
  line L232 (-5.9959, -15.9267) -> (-5.9984, -15.8868)
  line L233 (-6.0445, -15.9385) -> (-5.9959, -15.9267)
  line L234 (-5.9896, -15.9933) -> (-6.0396, -15.9908)
  line L235 (-5.9846, -16.033) -> (-5.9896, -15.9933)
  line L236 (-6.0324, -16.0478) -> (-5.9846, -16.033)
  line L237 (-5.9742, -16.099) -> (-6.0241, -16.0997)
  line L238 (-5.9667, -16.1383) -> (-5.9742, -16.099)
  line L239 (-6.0134, -16.156) -> (-5.9667, -16.1383)
  line L240 (-5.9521, -16.2035) -> (-6.0019, -16.2074)
  line L241 (-5.9421, -16.2423) -> (-5.9521, -16.2035)
  line L242 (-5.9877, -16.2629) -> (-5.9421, -16.2423)
  line L243 (-5.9235, -16.3065) -> (-5.973, -16.3134)
  line L244 (-5.9111, -16.3445) -> (-5.9235, -16.3065)
  line L245 (-5.9553, -16.368) -> (-5.9111, -16.3445)
  line L246 (-5.8885, -16.4074) -> (-5.9374, -16.4175)
  line L247 (-5.8737, -16.4446) -> (-5.8885, -16.4074)
  line L248 (-5.9163, -16.4708) -> (-5.8737, -16.4446)
  line L249 (-5.8472, -16.506) -> (-5.8954, -16.5191)
  line L250 (-5.8302, -16.5421) -> (-5.8472, -16.506)
  line L251 (-5.871, -16.571) -> (-5.8302, -16.5421)
  line L252 (-5.7998, -16.6017) -> (-5.8471, -16.6178)
  line L253 (-5.7805, -16.6368) -> (-5.7998, -16.6017)
  line L254 (-5.8195, -16.6681) -> (-5.7805, -16.6368)
  line L255 (-5.7465, -16.6943) -> (-5.7927, -16.7134)
  line L256 (-5.7251, -16.7281) -> (-5.7465, -16.6943)
  line L257 (-5.762, -16.7618) -> (-5.7251, -16.7281)
  line L258 (-5.6875, -16.7834) -> (-5.7324, -16.8053)
  line L259 (-5.664, -16.8157) -> (-5.6875, -16.7834)
  line L260 (-5.6987, -16.8517) -> (-5.664, -16.8157)
  line L261 (-5.623, -16.8685) -> (-5.6665, -16.8932)
  line L262 (-5.5975, -16.8994) -> (-5.623, -16.8685)
  line L263 (-5.6299, -16.9374) -> (-5.5975, -16.8994)
  line L264 (-5.5533, -16.9495) -> (-5.5952, -16.9769)
  line L265 (-5.5259, -16.9787) -> (-5.5533, -16.9495)
  line L266 (-5.5559, -17.0187) -> (-5.5259, -16.9787)
  line L267 (-5.4787, -17.0259) -> (-5.5187, -17.0559)
  line L268 (-5.4495, -17.0533) -> (-5.4787, -17.0259)
  line L269 (-5.4769, -17.0952) -> (-5.4495, -17.0533)
  line L270 (-5.3994, -17.0975) -> (-5.4374, -17.1299)
  line L271 (-5.3685, -17.123) -> (-5.3994, -17.0975)
  line L272 (-5.3932, -17.1665) -> (-5.3685, -17.123)
  line L273 (-5.3157, -17.164) -> (-5.3517, -17.1987)
  line L274 (-5.2834, -17.1875) -> (-5.3157, -17.164)
  line L275 (-5.3053, -17.2324) -> (-5.2834, -17.1875)
  line L276 (-5.2281, -17.2251) -> (-5.2618, -17.262)
  line L277 (-5.1943, -17.2465) -> (-5.2281, -17.2251)
  line L278 (-5.2134, -17.2927) -> (-5.1943, -17.2465)
  line L279 (-5.1368, -17.2805) -> (-5.1681, -17.3195)
  line L280 (-5.1017, -17.2998) -> (-5.1368, -17.2805)
  line L281 (-5.1178, -17.3471) -> (-5.1017, -17.2998)
  line L282 (-5.0421, -17.3302) -> (-5.071, -17.371)
  line L283 (-5.006, -17.3472) -> (-5.0421, -17.3302)
  line L284 (-5.0191, -17.3954) -> (-5.006, -17.3472)
  line L285 (-4.9446, -17.3737) -> (-4.9708, -17.4163)
  line L286 (-4.9074, -17.3885) -> (-4.9446, -17.3737)
  line L287 (-4.9175, -17.4374) -> (-4.9074, -17.3885)
  line L288 (-4.8445, -17.4111) -> (-4.868, -17.4553)
  line L289 (-4.8065, -17.4235) -> (-4.8445, -17.4111)
  line L290 (-4.8134, -17.473) -> (-4.8065, -17.4235)
  line L291 (-4.7423, -17.4421) -> (-4.7629, -17.4877)
  line L292 (-4.7035, -17.4521) -> (-4.7423, -17.4421)
  line L293 (-4.7074, -17.5019) -> (-4.7035, -17.4521)
  line L294 (-4.6383, -17.4667) -> (-4.656, -17.5134)
  line L295 (-4.599, -17.4742) -> (-4.6383, -17.4667)
  line L296 (-4.5997, -17.5241) -> (-4.599, -17.4742)
  line L297 (-4.533, -17.4846) -> (-4.5478, -17.5324)
  line L298 (-4.4933, -17.4896) -> (-4.533, -17.4846)
  line L299 (-4.4908, -17.5396) -> (-4.4933, -17.4896)
  line L300 (-4.4267, -17.4959) -> (-4.4385, -17.5445)
  line L301 (-4.3868, -17.4984) -> (-4.4267, -17.4959)
  line L302 (-4.3812, -17.5481) -> (-4.3868, -17.4984)
  dimension "d28" = 3.5
  dimension "d29" = 1
  dimension "d30" = 100
  dimension "d31" = 100
  dimension "d33" = 0.04
  dimension "d34" = 0.05
  dimension "d36" = 360
  constraint concentric A1 A2
  constraint concentric A2 A3
  constraint coincident A2 L2.start
  constraint coincident A2 L4.end
  constraint horizontal L3
  constraint midpoint L3 L5.start
  constraint vertical L5
  constraint coincident A1.centre A2.centre
  measures "d28" diameter of A2
  measures "d29" diameter of A3
  measures "d30" angle of L2 L3
  measures "d31" angle of L3 L4
  measures "d33" distance of L2.end L3.end
  measures "d34" distance of L3.end L4.end
extrude "Extruir6" add sketch "Boceto6" along normal blind 2.5 separate body contours A2 L2 L3 L4 L6 L7 L8 L9 L10 L11 L12 L13 L14 L15 L16 L17 L18 L19 L20 L21 L22 L23 L24 L25 L26 L27 L28 L29 L30 L31 L32 L33 L34 L35 L36 L37 L38 L39 L40 L41 L42 L43 L44 L45 L46 L47 L48 L49 L50 L51 L52 L53 L54 L55 L56 L57 L58 L59 L60 L61 L62 L63 L64 L65 L66 L67 L68 L69 L70 L71 L72 L73 L74 L75 L76 L77 L78 L79 L80 L81 L82 L83 L84 L85 L86 L87 L88 L89 L90 L91 L92 L93 L94 L95 L96 L97 L98 L99 L100 L101 L102 L103 L104 L105 L106 L107 L108 L109 L110 L111 L112 L113 L114 L115 L116 L117 L118 L119 L120 L121 L122 L123 L124 L125 L126 L127 L128 L129 L130 L131 L132 L133 L134 L135 L136 L137 L138 L139 L140 L141 L142 L143 L144 L145 L146 L147 L148 L149 L150 L151 L152 L153 L154 L155 L156 L157 L158 L159 L160 L161 L162 L163 L164 L165 L166 L167 L168 L169 L170 L171 L172 L173 L174 L175 L176 L177 L178 L179 L180 L181 L182 L183 L184 L185 L186 L187 L188 L189 L190 L191 L192 L193 L194 L195 L196 L197 L198 L199 L200 L201 L202 L203 L204 L205 L206 L207 L208 L209 L210 L211 L212 L213 L214 L215 L216 L217 L218 L219 L220 L221 L222 L223 L224 L225 L226 L227 L228 L229 L230 L231 L232 L233 L234 L235 L236 L237 L238 L239 L240 L241 L242 L243 L244 L245 L246 L247 L248 L249 L250 L251 L252 L253 L254 L255 L256 L257 L258 L259 L260 L261 L262 L263 L264 L265 L266 L267 L268 L269 L270 L271 L272 L273 L274 L275 L276 L277 L278 L279 L280 L281 L282 L283 L284 L285 L286 L287 L288 L289 L290 L291 L292 L293 L294 L295 L296 L297 L298 L299 L300 L301 L302 makes body 3
equation "d7 = ( d8 - d5 ) / 2"
equation "d12 = ( d11 - 19.8 mm ) / 2"
equation "d24 = 19.1 mm - 16.5 mm"
equation "d30 = d31"

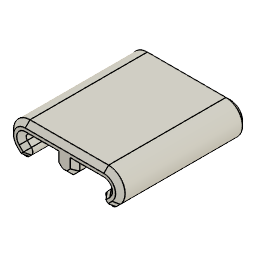
design "SEGUROS MOTORES 2"
Autodesk Fusion 360 part; units mm, degrees
sketch "Boceto1" plane through (0, 0, 0) normal (0, 1, 0) x (1, 0, 0)
  line L0 (-5.4, 0) -> (-6.5464, -1.1464)
  line L1 (-5.4, 0) -> (-3.3228, 0) construction
  line L2 (-6.1929, -2) -> (-1.75, -2)
  line L3 (-1.75, -2) -> (-1.75, 0)
  line L4 (0, -0.3508) -> (0, 0)
  line L5 (-5.4, 0) -> (0, 0)
  arc A0 (-6.5464, -1.1464) -> (-6.1929, -2) centre (-6.1929, -1.5) ccw
  line L6 (0.1, -0.3508) -> (0.1, 0.1)
  line L7 (-5.4414, 0.1) -> (0.1, 0.1)
  line L8 (-5.4414, 0.1) -> (-6.6172, -1.0757)
  arc A1 (-6.6172, -1.0757) -> (-6.1929, -2.1) centre (-6.1929, -1.5) ccw
  line L9 (-6.1929, -2.1) -> (-1.65, -2.1)
  line L10 (-1.65, -2.1) -> (-1.65, 0)
  line L11 (-5.4414, 0.1) -> (-6.8556, 1.5142)
  line L12 (-6.8556, 1.5142) -> (-8.0314, 0.3385)
  line L13 (-6.1929, -4.1) -> (0, -4.1)
  arc A2 (-8.0314, 0.3385) -> (-6.1929, -4.1) centre (-6.1929, -1.5) ccw
  line L14 (5.4414, 0.1) -> (6.8556, 1.5142)
  line L15 (5.4414, 0.1) -> (6.6172, -1.0757)
  arc A3 (6.1929, -2.1) -> (6.6172, -1.0757) centre (6.1929, -1.5) ccw
  line L16 (6.8556, 1.5142) -> (8.0314, 0.3385)
  arc A4 (6.1929, -4.1) -> (8.0314, 0.3385) centre (6.1929, -1.5) ccw
  line L17 (6.1929, -4.1) -> (0, -4.1)
  line L18 (6.1929, -2.1) -> (1.65, -2.1)
  line L19 (1.65, -2.1) -> (1.65, 0)
  line L20 (5.4, 0) -> (0, 0)
  point P0 (-7.4, -2)
  dimension "d1" = 135
  dimension "d2" = 3.5
  dimension "d3" = 2
  dimension "d5" = 10.8
  dimension "d6" = 0.5
  dimension "d7" = 0.1
  dimension "d8" = 2
  dimension "d9" = 2
  constraint horizontal L1
  constraint horizontal L2
  constraint perpendicular L2 L3
  constraint coincident L4.end L5.end
  constraint horizontal L5
  constraint coincident P0 L2
  constraint coincident P0 L0
  constraint tangent L2 A0
  constraint tangent L0 A0
  constraint coincident L3.end L5
  constraint perpendicular L8 L11
  constraint perpendicular L11 L12
  constraint horizontal L13
  constraint coincident L4 L13.end
  constraint tangent L12 A2
  constraint tangent L13 A2
  constraint symmetric L0.start L4 L20.start
  constraint symmetric L5.end L4 L20.end
  constraint symmetric L4 L7.start L14.start
  constraint symmetric L4 L8.end L15.end
  constraint symmetric L4 A1.end A3.start
  constraint symmetric L4 A1 A3
  constraint symmetric L4 L9.end L18.end
  constraint symmetric L4 L10.end L19.end
  constraint symmetric L4 L11.end L14.end
  constraint symmetric L4 L13.end L17.end
  constraint symmetric L4 L12.end L16.end
  constraint symmetric L4 L13.start A4.start
  constraint symmetric L4 A2 A4
  constraint coincident A0.centre A1.centre
  measures "d1" angle of L0 L1
  measures "d3" horizontal distance of L0.start P0
  measures "d6" radius of A0
  measures "d8" distance of L7.start L11.end
  measures "d9" distance of L9 L13
extrude "Extruir1" add sketch "Boceto1" along normal blind 20 contours L5 L8 A1 L9 L10 L11 L12 L13 A2 L14 L15 A3 L16 A4 L17 L18 L19 L20
fillet "Empalme1" radius 0.75 4 edges at (-5.4414, 10, -0.1) (-6.8556, 10, -1.5142) (5.4414, 10, -0.1) (6.8556, 10, -1.5142)
chamfer "Chaflán1" distance 1 angle 45 2 edges at (-1.65, 10, 0) (1.65, 10, 0)
chamfer "Chaflán2" distance 0.75 angle 45 2 faces at (0.55, 20, 3.4333) (0.55, 0, 3.4333)

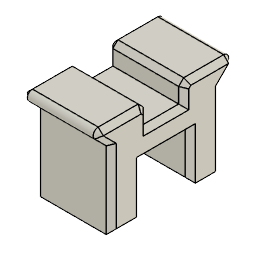
design "SEGUROS MOTORES"
Autodesk Fusion 360 part; units mm, degrees
sketch "Boceto1" plane through (0, 0, 0) normal (1, 0, 0) x (0, 1, 0)
  line L0 (2.4, 5.1) -> (2.4, 0)
  line L1 (2.4, 0) -> (5.4, 0)
  line L2 (5.4, 0) -> (5.4, 7.6)
  line L3 (0, 0) -> (0, 5.1)
  line L4 (0, 5.1) -> (2.4, 5.1)
  line L5 (5.4, 7.6) -> (6.5464, 8.7464)
  line L6 (5.4, 7.6) -> (9.5874, 7.6) construction
  line L7 (6.1929, 9.6) -> (2.25, 9.6)
  arc A0 (6.5464, 8.7464) -> (6.1929, 9.6) centre (6.1929, 9.1) ccw
  line L8 (-2.4, 5.1) -> (-2.4, 0)
  line L9 (-2.4, 0) -> (-5.4, 0)
  line L10 (-5.4, 0) -> (-5.4, 7.6)
  line L11 (0, 5.1) -> (-2.4, 5.1)
  line L12 (-5.4, 7.6) -> (-6.5464, 8.7464)
  arc A1 (-6.1929, 9.6) -> (-6.5464, 8.7464) centre (-6.1929, 9.1) ccw
  line L13 (-6.1929, 9.6) -> (-2.25, 9.6)
  line L14 (-1.75, 9.1) -> (-1.75, 7.6)
  line L15 (-1.75, 7.6) -> (1.75, 7.6)
  line L16 (1.75, 7.6) -> (1.75, 9.1)
  line L17 (-1.75, 9.1) -> (-2.25, 9.6)
  line L18 (1.75, 9.1) -> (2.25, 9.6)
  point P0 (7.4, 9.6)
  point P1 (-1.75, 9.6)
  point P2 (1.75, 9.6)
  dimension "d4" = 5.1
  dimension "d5" = 4.8
  dimension "d6" = 3
  dimension "d7" = 45
  dimension "d8" = 2
  dimension "d10" = 0.5
  dimension "d13" = 3.5
  dimension "d14" = 3.5
  dimension "d15" = 2
  dimension "d16" = 0.5
  dimension "d17" = 0.5
  dimension "d18" = 0.5
  dimension "d19" = 0.5
  dimension "d22" = 2.5
  constraint coincident L3.start origin
  constraint vertical L3
  constraint perpendicular L0 L4
  constraint coincident L3.start L1
  constraint horizontal L1
  constraint horizontal L6
  constraint horizontal L7
  constraint coincident P0 L5
  constraint coincident P0 L7
  constraint tangent L5 A0
  constraint tangent L7 A0
  constraint symmetric L0.start L3 L8.start
  constraint symmetric L0.end L3 L8.end
  constraint symmetric L1.end L3 L9.end
  constraint symmetric L2.end L3 L10.end
  constraint symmetric L4.start L3 L11.start
  constraint symmetric L3 L5.end L12.end
  constraint symmetric L3 L7.start A1.start
  constraint symmetric L3 A0 A1
  constraint perpendicular L13 L14
  constraint perpendicular L14 L15
  constraint perpendicular L7 L16
  constraint coincident P1 L14
  constraint coincident L13 P1
  constraint coincident P2 L16
  constraint coincident L7 P2
  measures "d4" distance of L3.start L3.end
  measures "d6" distance of L0 L2
  measures "d7" angle of L5 L6
  measures "d8" horizontal distance of L2.end P0
  measures "d10" radius of A0
  measures "d14" distance of L14.end L15.end
  measures "d15" distance of L7 L15
  measures "d16" distance of P1 L14.start
  measures "d17" distance of P1 L13.end
  measures "d18" distance of P2 L16.end
  measures "d19" distance of P2 L7.end
  measures "d22" distance of L11 L15
extrude "Extruir1" add sketch "Boceto1" along normal blind 7.5
chamfer "Chaflán1" distance 0.5 angle 45 2 faces at (7.5, -4.4, 4.2333) (0, -4.4, 4.2333)
chamfer "Chaflán2" distance 1 angle 45 2 edges at (3.75, 2.4, 0) (3.75, -2.4, 0)
equation "d14 = d13"
equation "d17 = d16"
equation "d19 = d18"

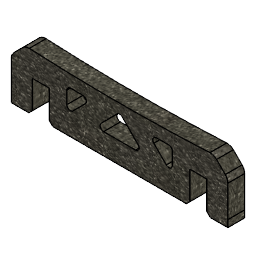
design "SOPORTE SUPERIOR"
Autodesk Fusion 360 part; units mm, degrees